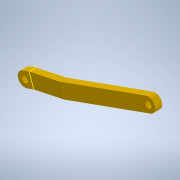
# Autodesk Inventor part: Dedo_3
Saved by Autodesk Inventor 2020 (Build 240168000, 168)
## iProperties
Created: 2021-07-29
Part Number: Dedo_3
Material: Generic
Document SubType Name: Modeling
Designer: chalo
Density: 1 g/cm^3
Appearance: Gold
Author: chalo
Autodesk Inventor part; units mm, degrees
ref_plane "YZ Plane" through (0, 0, 0) normal (1, 0, 0) x (0, 1, 0)
ref_plane "XZ Plane" through (0, 0, 0) normal (0, 1, 0) x (-1, 0, 0)
ref_plane "XY Plane" through (0, 0, 0) normal (0, 0, 1) x (1, 0, 0)
sketch "Sketch1" plane through (0, 0, 0) normal (0, 0, 1) x (1, 0, 0)
  circle A0 centre (1.6652, -2.7344) radius 1.1 projected
  circle A1 centre (1.6652, -2.7344) radius 2.5
  circle A2 centre (48.2864, 14.0238) radius 1.1 construction
  point P0 (0, 0)
  dimension "d0" = 5
  constraints: 1 centre point, 1 coincident
  measures "d0" diameter of A1
extrude "Extrusion1" add sketch "Sketch1" along normal blind 2.5
sketch "Sketch2" plane through (1.6652, -2.7344, 2.5) normal (0, 0, 1) x (1, 0, 0)
  circle A0 centre (0, 0) radius 2.5 projected
  circle A1 centre (0, 0) radius 1.1 projected
  circle A2 centre (46.6212, 16.7582) radius 1.1 projected
  circle A3 centre (46.6212, 16.7582) radius 2.5
  circle A4 centre (0, 0) radius 2.5 projected
  line L0 (0.8457, -2.3526) -> (47.4669, 14.4056)
  line L1 (-0.8457, 2.3526) -> (45.7756, 19.1109)
  point P0 (-1.6652, 2.7344)
  point P1 (0.8457, -2.3526)
  dimension "d4" = 5
  constraints: 4 end point, 4 point on circle, 4 tangent, 1 centre point, 1 coincident
  measures "d4" diameter of A3
extrude "Extrusion2" add sketch "Sketch2" along normal blind 2.5
sketch "Sketch3" plane through (0.8195, -0.3818, 5) normal (-0.3382652, 0.9410508, 0) x (0.9410508, 0.3382652, 0)
  line L0 (49.5417, 2.5) -> (0, 2.5) projected
  line L1 (0, 2.5) -> (0, 0) projected
  line L2 (49.5417, 0) -> (0, 0) projected
  line L3 (49.5417, 2.5) -> (49.5417, 0) projected
  line L4 (0, 2.5) -> (0, 2.5) projected
  line L5 (0, 2.5) -> (0, 0) projected
  line L6 (0, 0) -> (0, 0) projected
  line L7 (0, 2.5) -> (0, 0) projected
  line L8 (-2.5, 5) -> (2.5, 5) projected
  line L9 (-2.5, 0) -> (0, 0) projected
  line L10 (-2.5, 5) -> (-2.5, 0) projected
  line L11 (-2.5, 5) -> (2.5, 5) projected
  line L12 (2.5, 5) -> (16.6782, 2.5)
  line L13 (0, 2.5) -> (49.5417, 2.5) projected
  line L14 (2.5, 5) -> (2.5, 2.5) projected
  line L15 (0, 0) -> (49.5417, 0) projected
  line L16 (0, 2.5) -> (2.5, 2.5) projected
  line L17 (16.6782, 0) -> (2.5, 2.5)
  point P0 (-0.6421, 5)
  point P1 (16.6782, 2.5)
  dimension "d7" = 10
  constraints: 4 end point, 2 point on line, 1 vertical alignment
  measures "d7" angle of L0 L12
extrude "Extrusion3" add sketch "Sketch3" against normal blind 5 contours L0 L14 L12
sketch "Sketch4" plane through (3.1722, 0.4639, 0) normal (-0.9410508, -0.3382652, 0) x (0, 0, 1)
  line L0 (0, -2.5) -> (2.5, -2.5) projected
  line L1 (2.5, 0) -> (2.5, -2.5) projected
  line L2 (0, 0) -> (2.5, 0) projected
  line L3 (0, 0) -> (0, -2.5) projected
  line L4 (0, -2.5) -> (0, -5) projected
  line L5 (2.5, -5) -> (0, -5) projected
  line L6 (2.5, -2.5) -> (2.5, -5) projected
  point P0 (0, 0.6365)
extrude "Extrusion4" add sketch "Sketch4" along normal up to surface
sketch "Sketch5" plane through (0.8195, -0.3818, 5) normal (-0.3382652, 0.9410508, 0) x (0.9410508, 0.3382652, 0)
  line L0 (0, 5) -> (0, 0) projected
  line L1 (0, 0) -> (0, 0) projected
  line L2 (0, 5) -> (0, 0) projected
  line L3 (0, 5) -> (0, 5) projected
  line L4 (49.5417, 2.5) -> (16.6782, 2.5) projected
  line L5 (16.6782, 2.5) -> (2.5, 5) projected
  line L6 (2.5, 5) -> (0, 5) projected
  line L7 (0, 5) -> (0, 0) projected
  line L8 (49.5417, 0) -> (0, 0) projected
  line L9 (49.5417, 2.5) -> (49.5417, 0) projected
  line L10 (-1.1, 0) -> (-1.1, 5) projected
  line L11 (-2.5, 5) -> (-2.5, 0) projected
  line L12 (-2.5, 0) -> (0, 0) projected
  line L13 (-2.5, 5) -> (0, 5) projected
  line L14 (-2.5, 2.5) -> (2.5, 2.5)
  line L15 (2.5, 2.5) -> (16.6782, 0)
  point P0 (-0.6421, 5)
  constraints: 4 end point, 2 vertical alignment, 1 horizontal, 1 midpoint, 1 point on line
extrude "Extrusion5" cut sketch "Sketch5" against normal up to next contours L14 L15 L8 L0 | L0 L12 L10 L14 | L10 L12 L11 L14
body "Solid1"
